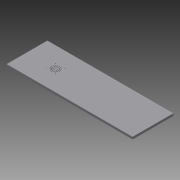
# Autodesk Inventor part: placa verticala pompa vid
Saved by Autodesk Inventor 2015 SP1 (Build 190203100, 203)
## iProperties
Created: 2015-08-10
Part Number: placa verticala pompa vid
Material: Generic
Document SubType Name: Modeling
Designer: ubik
Density: 1 g/cm^3
Appearance: Default
Author: ubik
Autodesk Inventor part; units mm, degrees
ref_plane "YZ Plane" through (0, 0, 0) normal (1, 0, 0) x (0, 1, 0)
ref_plane "XZ Plane" through (0, 0, 0) normal (0, 1, 0) x (-1, 0, 0)
ref_plane "XY Plane" through (0, 0, 0) normal (0, 0, 1) x (1, 0, 0)
sketch "Sketch1" plane through (0, 0, 0) normal (0, 0, 1) x (1, 0, 0)
  line L0 (-222.5, 72) -> (222.5, 72)
  line L1 (222.5, 72) -> (222.5, -72)
  line L2 (222.5, -72) -> (-222.5, -72)
  line L3 (-222.5, -72) -> (-222.5, 72)
  point P0 (0, 0)
  dimension "d0" = 445
  dimension "d1" = 144
  dimension "d2" = 72
  dimension "d3" = 222.5
  constraints: 8 end point, 2 parallel, 1 horizontal, 1 perpendicular
  measures "d0" distance of L1.end L2.end
  measures "d1" distance of L0.end L1.end
  measures "d2" distance from line of point (0, 0) L0
  measures "d3" distance from line of point (0, 0) L3
extrude "Extrusion1" add sketch "Sketch1" along normal blind 8
hole "Hole1" at (-137.5, 16, 8) direction (0, 0, -1) diameter 3 end through all
pattern_linear "Rectangular Pattern1" count 2 spacing 32 along (0, -1, 0) count 2 spacing 32 along (1, 0, 0) of "Hole1"
sketch "Sketch2" plane through (0, 0, 8) normal (0, 0, 1) x (1, 0, 0)
  circle A0 centre (-121.5, 0) radius 1.5
  line L0 (-222.5, 72) -> (-222.5, -72) projected
  circle A1 centre (-121.5, 6) radius 1.5
  circle A2 centre (-126.6962, 3) radius 1.5
  circle A3 centre (-126.6962, -3) radius 1.5
  circle A4 centre (-121.5, -6) radius 1.5
  circle A5 centre (-116.3038, -3) radius 1.5
  circle A6 centre (-116.3038, 3) radius 1.5
  circle A7 centre (-121.5, 10) radius 1.5
  circle A8 centre (-126.5, 8.6603) radius 1.5
  circle A9 centre (-130.1603, 5) radius 1.5
  circle A10 centre (-131.5, 0) radius 1.5
  circle A11 centre (-130.1603, -5) radius 1.5
  circle A12 centre (-126.5, -8.6603) radius 1.5
  circle A13 centre (-121.5, -10) radius 1.5
  circle A14 centre (-116.5, -8.6603) radius 1.5
  circle A15 centre (-112.8397, -5) radius 1.5
  circle A16 centre (-111.5, 0) radius 1.5
  circle A17 centre (-112.8397, 5) radius 1.5
  circle A18 centre (-116.5, 8.6603) radius 1.5
  circle A19 centre (-121.5, 14) radius 1.5
  circle A20 centre (-126.8576, 12.9343) radius 1.5
  circle A21 centre (-131.3995, 9.8995) radius 1.5
  circle A22 centre (-134.4343, 5.3576) radius 1.5
  circle A23 centre (-135.5, 0) radius 1.5
  circle A24 centre (-134.4343, -5.3576) radius 1.5
  circle A25 centre (-131.3995, -9.8995) radius 1.5
  circle A26 centre (-126.8576, -12.9343) radius 1.5
  circle A27 centre (-121.5, -14) radius 1.5
  circle A28 centre (-116.1424, -12.9343) radius 1.5
  circle A29 centre (-111.6005, -9.8995) radius 1.5
  circle A30 centre (-108.5657, -5.3576) radius 1.5
  circle A31 centre (-107.5, 0) radius 1.5
  circle A32 centre (-108.5657, 5.3576) radius 1.5
  circle A33 centre (-111.6005, 9.8995) radius 1.5
  circle A34 centre (-116.1424, 12.9343) radius 1.5
  point P0 (0, 0)
  dimension "d21" = 3
  dimension "d22" = 101
  dimension "d23" = 3
  dimension "d24" = 6
  dimension "d27" = 360
  dimension "d29" = 3
  dimension "d30" = 10
  dimension "d33" = 360
  dimension "d35" = 3
  dimension "d36" = 14
  dimension "d39" = 360
  constraints: 35 centre point, 2 coincident, 81 other
  measures "d21" diameter of A0
  measures "d22" distance from line of A0.centre L0
  measures "d23" diameter of A1
  measures "d24" distance of A0.centre A1.centre
  measures "d29" diameter of A7
  measures "d30" distance of A0.centre A7.centre
  measures "d35" diameter of A19
  measures "d36" distance of A0.centre A19.centre
extrude "Extrusion2" cut sketch "Sketch2" against normal through all
equation "\"d2\" = 0.5 * d1"
equation "\"d3\" = 0.5 * d0"
body "Solid1"
